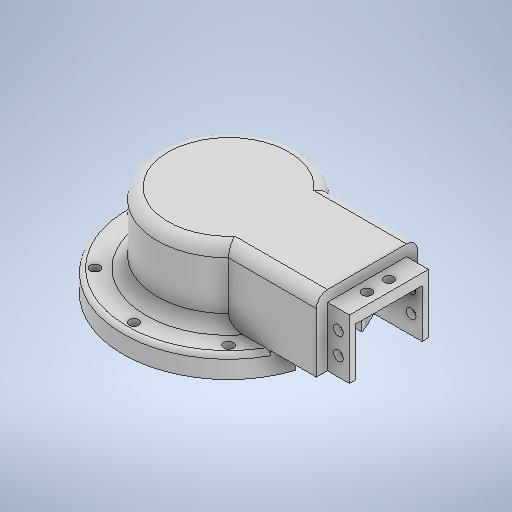
# Autodesk Inventor part: pulley_case_part_1
Saved by Autodesk Inventor 2025 (Build 290162000, 162)
## iProperties
Created: 2025-01-31
Part Number: pulley_case_part_1
Material: Generic
Document SubType Name: Modeling
Designer: danielrachi
Density: 1 g/cm^3
Appearance: Default
Author: danielrachi
Autodesk Inventor part; units mm, degrees
ref_plane "YZ Plane" through (0, 0, 0) normal (1, 0, 0) x (0, 1, 0)
ref_plane "XZ Plane" through (0, 0, 0) normal (0, 1, 0) x (-1, 0, 0)
ref_plane "XY Plane" through (0, 0, 0) normal (0, 0, 1) x (1, 0, 0)
sketch "Sketch1" plane through (0, 0, 0) normal (0, 1, 0) x (-1, 0, 0)
  circle A0 centre (0, 0) radius 27.5
  circle A1 centre (0, 0) radius 48
  circle A2 centre (0, -43) radius 2.25
  circle A3 centre (30.4056, -30.4056) radius 2.25
  circle A4 centre (43, 0) radius 2.25
  circle A5 centre (30.4056, 30.4056) radius 2.25
  circle A6 centre (0, 43) radius 2.25
  circle A7 centre (-30.4056, 30.4056) radius 2.25
  circle A8 centre (-43, 0) radius 2.25
  circle A9 centre (-30.4056, -30.4056) radius 2.25
  dimension "d0" = 55
  dimension "d1" = 96
  dimension "d3" = 4.5
  dimension "d4" = 43
  dimension "d7" = 360
  constraints: 10 centre point, 2 coincident, 1 vertical alignment, 17 other
  measures "d0" diameter of A0
  measures "d1" diameter of A1
  measures "d3" diameter of A2
  measures "d4" distance of A2.centre point (0, 0)
extrude "Extrusion1" add sketch "Sketch1" along normal blind 10 contours A1 | A8
sketch "Sketch2" plane through (0, 10, 0) normal (0, 1, 0) x (1, 0, 0)
  circle A0 centre (0, 0) radius 32.5
  circle A1 centre (0, 0) radius 27.5
  line L0 (22.981, 22.981) -> (22.981, -22.981)
  line L1 (0, 0) -> (22.981, -22.981)
  line L2 (0, 0) -> (32.5, 0) construction
  point P0 (22.981, 0)
  point P1 (22.981, -15.1038)
  point P2 (22.981, 15.1038)
  point P3 (19.4454, -19.4454)
  dimension "d11" = 65
  dimension "d12" = 55
  dimension "d50" = 45
  constraints: 6 end point, 2 centre point, 2 coincident, 2 point on circle, 1 equal length, 1 horizontal, 1 midpoint, 1 vertical
  measures "d11" diameter of A0
  measures "d12" diameter of A1
  measures "d50" angle of L1 L2
extrude "Extrusion2" add sketch "Sketch2" along normal blind 22 contours L0 A1 L1 A0 | L1 A1 L0
sketch "Sketch17" plane through (0, 10, 0) normal (0, 1, 0) x (1, 0, 0)
  line L0 (22.981, -15.1038) -> (22.981, -22.981) projected
  line L1 (22.981, -15.1038) -> (48, -15.1038)
  line L2 (48, -15.1038) -> (48, 15.1038)
  line L3 (48, 15.1038) -> (22.981, 15.1038)
  line L4 (22.981, 15.1038) -> (22.981, -15.1038)
  circle A0 centre (0, 0) radius 48 projected
  point P0 (45.5618, -15.1038)
  point P1 (45.5618, 15.1038)
  constraints: 8 end point, 2 parallel, 1 coincident, 1 horizontal, 1 perpendicular, 1 tangent
extrude "Extrusion14" cut sketch "Sketch17" against normal up to next contours L4 L3 A0 L1 picked at (31.3207, 0)
sketch "Sketch18" plane through (0, 32, 0) normal (0, 1, 0) x (1, 0, 0)
  arc A0 (22.981, 22.981) -> (22.981, -22.981) centre (0, 0) ccw projected
  circle A1 centre (0, 0) radius 32.5
  arc A2 (22.981, 15.1038) -> (22.981, -15.1038) centre (0, 0) ccw projected
  line L0 (22.981, 22.981) -> (22.981, -22.981)
  point P0 (22.981, -15.1038)
  point P1 (22.981, 15.1038)
  constraints: 2 end point, 1 coincident, 1 vertical, 3 other
extrude "Extrusion15" add sketch "Sketch18" along normal blind 10 contours L0 A2 A0 | L0 A2
sketch "Sketch19" plane through (22.981, 10, -15.1038) normal (1, 0, 0) x (0, 0, -1)
  line L0 (-30.2076, 0) -> (-38.0848, 0) projected
  line L1 (-38.0848, 32) -> (7.8772, 32) projected
  line L2 (-38.0848, 0) -> (-38.0848, 32)
  line L3 (-38.0848, 32) -> (7.8772, 32)
  line L4 (7.8772, 32) -> (7.8772, 0)
  line L5 (0, 0) -> (0, 22) projected
  line L6 (7.8772, 0) -> (0, 0)
  line L7 (0, 0) -> (0, 22)
  line L8 (-30.2076, 0) -> (-30.2076, 22) projected
  line L9 (0, 22) -> (-30.2076, 22)
  line L10 (-30.2076, 22) -> (-30.2076, 0)
  line L11 (-30.2076, 0) -> (-38.0848, 0)
  point P0 (-15.1038, -10)
  constraints: 16 end point, 7 perpendicular, 1 vertical
extrude "Extrusion16" add sketch "Sketch19" along normal blind 50
sketch "Sketch20" plane through (72.981, 10, -15.1038) normal (1, 0, 0) x (0, 0, -1)
  line L0 (-47.6038, 0) -> (17.3962, 0) projected
  line L1 (-33.0848, 0) -> (2.8772, 0)
  line L2 (2.8772, 0) -> (2.8772, 27)
  line L3 (2.8772, 27) -> (-33.0848, 27)
  line L4 (-33.0848, 27) -> (-33.0848, 0)
  line L5 (-38.0848, 32) -> (-38.0848, 0) projected
  line L6 (7.8772, 0) -> (7.8772, 32) projected
  line L7 (7.8772, 32) -> (-38.0848, 32) projected
  point P0 (-15.1038, -10)
  point P1 (2.8772, 0)
  dimension "d67" = 5
  dimension "d68" = 5
  dimension "d69" = 5
  constraints: 8 end point, 2 parallel, 1 horizontal, 1 perpendicular, 1 point on line
  measures "d67" distance between parallel lines of L5 L4
  measures "d68" distance between parallel lines of L6 L2
  measures "d69" distance between parallel lines of L3 L7
extrude "Extrusion17" cut sketch "Sketch20" against normal blind 10 contours L5 L7 L6 L0 L2 L3 L4
sketch "Sketch21" plane through (72.981, 37, 17.981) normal (0, 1, 0) x (1, 0, 0)
  line L0 (0, 2.8772) -> (0, 33.0848) projected
  line L1 (0, 17.981) -> (-10, 17.981)
  line L2 (-10, -5) -> (-10, 40.9619) projected
  circle A0 centre (-5, 22.981) radius 2.25
  circle A1 centre (-5, 12.981) radius 2.25
  point P0 (-72.981, 17.981)
  point P1 (-5, 17.981)
  dimension "d72" = 4.5
  dimension "d73" = 5
  constraints: 3 midpoint, 2 centre point, 2 end point, 1 symmetric about line, 1 vertical alignment, 1 other
  measures "d72" diameter of A0
  measures "d73" distance from line of A0.centre L1
extrude "Extrusion18" cut sketch "Sketch21" against normal blind 50
sketch "Sketch22" plane through (72.981, 10, 17.981) normal (0, 0, 1) x (1, 0, 0)
  line L0 (0, 0) -> (0, 27) projected
  line L1 (0, 13.5) -> (-10, 13.5)
  line L2 (-10, 32) -> (-10, 0) projected
  circle A0 centre (-5, 18.5) radius 2.25
  circle A1 centre (-5, 8.5) radius 2.25
  point P0 (-72.981, -10)
  point P1 (-5, 13.5)
  dimension "d76" = 4.5
  dimension "d77" = 5
  constraints: 2 centre point, 2 end point, 2 midpoint, 1 horizontal, 1 point on line, 1 symmetric about line, 1 vertical alignment, 1 other
  measures "d76" diameter of A0
  measures "d77" distance of point (-5, 13.5) A0.centre
extrude "Extrusion19" cut sketch "Sketch22" against normal blind 50
fillet "Fillet5" radius 5 3 edges at (-32.5, 42, 0) (42.981, 42, 22.981) (42.981, 42, -22.981)
fillet "Fillet6" radius 5 1 edges at (-32.5, 10, 0)
fillet "Fillet7" radius 2 1 edges at (-48, 10, 0)
equation "\"d0\" = pulley_diameter"
equation "\"d1\" = motor_diameter"
equation "\"d9\" = thickness"
equation "\"d11\" = pulley_diameter + thickness"
equation "\"d12\" = pulley_diameter"
equation "\"d13\" = pulley_width - thickness"
equation "\"d60\" = pulley_width - thickness"
equation "\"d63\" = thickness"
equation "\"d67\" = 0.5 * thickness"
equation "\"d68\" = 0.5 * thickness"
equation "\"d69\" = 0.5 * thickness"
equation "\"d70\" = thickness"
equation "\"pulley_diameter\" = 55"
equation "\"motor_diameter\" = 96"
equation "\"pulley_width\" = 32"
equation "\"thickness\" = 10"
equation "\"belt_perimeter\" = 582.5"
equation "\"belt_pulley_half_perimeter\" = 138.23"
equation "\"belt_pulley_to_pulley_perimeter\" = belt_perimeter - 2 * belt_pulley_half_perimeter"
equation "\"pulley_separation\" = -belt_pulley_half_perimeter + 0.5 * belt_perimeter"
body "Solid1"
